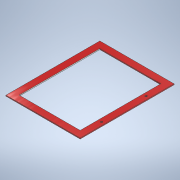
# Autodesk Inventor part: Tapa Superior
Saved by Autodesk Inventor 2022.6 (Build 266554000, 554)
## iProperties
Created: 2025-01-14
Part Number: Tapa Superior
Material: Genérico
Document SubType Name: Modeling
Designer: johan
Density: 1 g/cm^3
Appearance: Valor por defecto
Author: johan
Autodesk Inventor part; units mm, degrees
ref_plane "YZ Plane" through (0, 0, 0) normal (1, 0, 0) x (0, 1, 0)
ref_plane "XZ Plane" through (0, 0, 0) normal (0, 1, 0) x (-1, 0, 0)
ref_plane "XY Plane" through (0, 0, 0) normal (0, 0, 1) x (1, 0, 0)
sketch "Boceto1" plane through (0, 0, 0) normal (0, 1, 0) x (-1, 0, 0)
  line L0 (0, 0) -> (180, 0)
  line L1 (180, 0) -> (180, -240)
  line L2 (180, -240) -> (0, -240)
  line L3 (0, -240) -> (0, 0)
  line L4 (-3, -243) -> (183, -243)
  line L5 (183, -243) -> (183, 3)
  line L6 (183, 3) -> (-3, 3)
  line L7 (-3, 3) -> (-3, -243)
  line L8 (203, 23) -> (203, -263)
  line L9 (203, -263) -> (-23, -263)
  line L10 (-23, -263) -> (-23, 23)
  line L11 (-23, 23) -> (203, 23)
  dimension "d0" = 180
  dimension "d1" = 240
  dimension "d2" = 3
  dimension "d5" = 20
  constraints: 24 end point, 6 parallel, 3 perpendicular, 1 horizontal, 6 other
  measures "d0" distance of L1.end L2.end
  measures "d1" distance of L0.end L1.end
  measures "d2" distance between parallel lines of L2 L4
  measures "d5" distance between parallel lines of L5 L8
extrude "Extrusión3" add sketch "Boceto1" along normal blind 3 contours L8 L9 L10 L11
sketch "Boceto6" plane through (0, 3, 0) normal (0, 1, 0) x (1, 0, 0)
  line L0 (-183, -3) -> (-183, 243) projected
  line L1 (-183, 243) -> (3, 243) projected
  line L2 (3, 243) -> (3, -3) projected
  line L3 (3, -3) -> (-183, -3) projected
  line L4 (-203, 263) -> (-203, -23) projected
  line L5 (-203, -23) -> (23, -23) projected
  line L6 (23, -23) -> (23, 263) projected
  line L7 (23, 263) -> (-203, 263) projected
  line L8 (23, 91.3088) -> (23, 114.6899)
  line L9 (3, 114.6899) -> (3, 91.3088)
  circle A0 centre (13, 188) radius 3.175
  circle A1 centre (13, 52) radius 3.175
  point P0 (0, 0)
  dimension "d32" = 6.35
  dimension "d33" = 75
  dimension "d34" = 6.35
  dimension "d35" = 75
  constraints: 4 end point, 2 centre point, 2 point on line, 1 parallel
  measures "d32" diameter of A0
  measures "d33" distance from line of L7 A0.centre
  measures "d34" diameter of A1
  measures "d35" distance from line of L5 A1.centre
extrude "Extrusión8" cut sketch "Boceto6" against normal blind 3 contours A0 | A1
